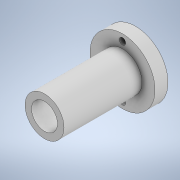
# Autodesk Inventor part: RD005_ペンホルダ
Saved by Autodesk Inventor 2021 (Build 250183000, 183)
## iProperties
Created: 2020-10-26
Part Number: RD005_ペンホルダ
Material: 一般
Document SubType Name: Modeling
Designer: ryusei
Density: 1 g/cm^3
Appearance: 既定
Author: ryusei
Autodesk Inventor part; units mm, degrees
ref_plane "YZ Plane" through (0, 0, 0) normal (1, 0, 0) x (0, 1, 0)
ref_plane "XZ Plane" through (0, 0, 0) normal (0, 1, 0) x (-1, 0, 0)
ref_plane "XY Plane" through (0, 0, 0) normal (0, 0, 1) x (1, 0, 0)
sketch "スケッチ1" plane through (0, 0, 0) normal (0, 0, 1) x (1, 0, 0)
  circle A0 centre (0, 0) radius 12.5
  dimension "d0" = 25
  constraints: 1 centre point, 1 coincident
  measures "d0" diameter of A0
extrude "押し出し1" add sketch "スケッチ1" along normal blind 5
sketch "スケッチ2" plane through (0, 0, 5) normal (0, 0, 1) x (1, 0, 0)
  circle A0 centre (0, 0) radius 7.5
  dimension "d3" = 15
  constraints: 1 centre point, 1 coincident
  measures "d3" diameter of A0
extrude "押し出し2" add sketch "スケッチ2" along normal blind 30
sketch "スケッチ3" plane through (0, 0, 35) normal (0, 0, 1) x (1, 0, 0)
  point P0 (0, 0)
hole "穴1" at (0, 0, 35) direction (0, 0, -1) diameter 10 end through all
sketch "スケッチ4" plane through (0, 0, 5) normal (0, 0, 1) x (1, 0, 0)
  circle A0 centre (0, 0) radius 5 projected
  line L0 (0, 0) -> (12.5, 0) construction
  circle A1 centre (0, 0) radius 12.5 projected
  point P0 (0, 10)
  point P1 (0, -10)
  dimension "d13" = 20
  constraints: 2 end point, 1 horizontal, 1 horizontal alignment, 1 symmetric about line, 1 vertical alignment, 1 other
  measures "d13" distance of point (0, -10) point (0, 10)
hole "穴2" at (0, 10, 5) at (0, -10, 5) direction (0, 0, -1) diameter 2.459 end through all thread size "M3x0.5" class "6H" standard "ISO Metric profile"
